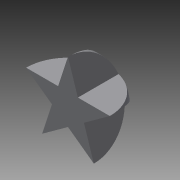
# Autodesk Inventor part: star
Saved by Autodesk Inventor 2013 (Build 170138000, 138)
## iProperties
Created: 2014-05-08
Part Number: star
Material: 一般
Document SubType Name: Modeling
Designer: andou
Density: 1 g/cm^3
Author: andou
Autodesk Inventor part; units mm, degrees
ref_plane "YZ Plane" through (0, 0, 0) normal (1, 0, 0) x (0, 1, 0)
ref_plane "XZ Plane" through (0, 0, 0) normal (0, 1, 0) x (-1, 0, 0)
ref_plane "XY Plane" through (0, 0, 0) normal (0, 0, 1) x (1, 0, 0)
sketch "スケッチ1" plane through (0, 0, 0) normal (0, 0, 1) x (1, 0, 0)
  arc A0 (13, 0) -> (0, 13) centre (0, 0) ccw
  line L0 (0, 0) -> (13, 0)
  line L1 (0, 13) -> (0, 0)
  point P0 (0, 0)
  dimension "d0" = 26
  constraints: 4 end point, 2 point on circle, 1 centre point, 1 coincident, 1 horizontal, 1 perpendicular
  measures "d0" diameter of A0
revolve "回転1" add sketch "スケッチ1" angle 360 about axis through (0, 13, 0) along (0, -1, 0)
sketch "スケッチ3" plane through (0, 0, 0) normal (0, -1, 0) x (1, 0, 0)
  circle A0 centre (0, 0) radius 13 projected
  line L0 (12.3637, 4.0172) -> (4.7225, -1.5344)
  line L1 (0, -4.9656) -> (-7.6412, -10.5172)
  line L2 (7.6412, -10.5172) -> (0, -4.9656)
  line L3 (-4.7225, -1.5344) -> (-12.3637, 4.0172)
  line L4 (0, 13) -> (-2.9187, 4.0172)
  line L5 (-4.7225, -1.5344) -> (-7.6412, -10.5172)
  line L6 (12.3637, 4.0172) -> (2.9187, 4.0172)
  line L7 (-2.9187, 4.0172) -> (-12.3637, 4.0172)
  line L8 (0, 13) -> (2.9187, 4.0172)
  line L9 (4.7225, -1.5344) -> (7.6412, -10.5172)
  constraints: 20 end point, 1 coincident, 1 vertical alignment, 7 other
extrude "押し出し2" cut sketch "スケッチ3" against normal blind 13 contours L0 L9 L2 L1 L5 L3 L7 L4 L8 L6 keep common part
